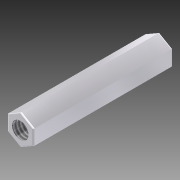
# Autodesk Inventor part: Stand-Off Posts 1inch
Saved by Autodesk Inventor 2012 (Build 160160000, 160)
## iProperties
Created: 2012-11-03
Part Number: Stand-Off Posts 1inch
Material: Default
Document SubType Name: Modeling
Designer: Rob
Density: 1 g/cm^3
Author: Rob
Autodesk Inventor part; units mm, degrees
ref_plane "YZ Plane" through (0, 0, 0) normal (1, 0, 0) x (0, 1, 0)
ref_plane "XZ Plane" through (0, 0, 0) normal (0, 1, 0) x (-1, 0, 0)
ref_plane "XY Plane" through (0, 0, 0) normal (0, 0, 1) x (1, 0, 0)
sketch "Sketch1" plane through (0, 0, 0) normal (0, 0, 1) x (1, 0, 0)
  line L0 (2.3812, -1.3748) -> (0, -2.7496)
  line L1 (0, -2.7496) -> (-2.3812, -1.3748)
  line L2 (-2.3812, -1.3748) -> (-2.3813, 1.3748)
  line L3 (-2.3813, 1.3748) -> (0, 2.7496)
  line L4 (0, 2.7496) -> (2.3812, 1.3748)
  line L5 (2.3812, 1.3748) -> (2.3812, -1.3748)
  circle A0 centre (0, 0) radius 1.4986
  point P0 (2.3812, 0)
  dimension "d1" = 2.9972
  constraints: 12 end point, 1 centre point, 1 coincident, 1 midpoint, 13 other
  measures "d1" diameter of A0
extrude "Extrusion1" add sketch "Sketch1" along normal blind 25.4
fillet "Fillet1" radius 0.254 5 edges at (2.3812, 0, 0) (1.1906, -2.0622, 0) (-1.1906, -2.0622, 0) (-1.1906, 2.0622, 0) (1.1906, 2.0622, 0)
fillet "Fillet2" radius 0.254 6 edges at (2.3812, 0, 25.4) (1.1906, 2.0622, 25.4) (-1.1906, 2.0622, 25.4) (-2.3812, 0, 25.4) (-1.1906, -2.0622, 25.4) (1.1906, -2.0622, 25.4)
thread "Thread1" size "5-40 UNC" class "2B" standard "ANSI Unified Screw Threads" full length
body "Solid1"
